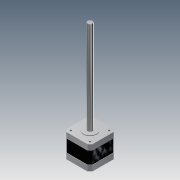
# Autodesk Inventor part: StepperDrive
Saved by Autodesk Inventor 2014 (Build 180170000, 170)
## iProperties
Created: 2014-08-06
Part Number: StepperDrive
Material: Generic
Document SubType Name: Modeling
Designer: Peele
Density: 1 g/cm^3
Appearance: Chrome - Polished
Author: Peele
Autodesk Inventor part; units mm, degrees
ref_plane "YZ Plane" through (0, 0, 0) normal (1, 0, 0) x (0, 1, 0)
ref_plane "XZ Plane" through (0, 0, 0) normal (0, 1, 0) x (-1, 0, 0)
ref_plane "XY Plane" through (0, 0, 0) normal (0, 0, 1) x (1, 0, 0)
sketch "Sketch1" plane through (0, 0, 0) normal (0, 0, 1) x (1, 0, 0)
  line L0 (-21.15, -21.15) -> (21.15, -21.15)
  line L1 (21.15, -21.15) -> (21.15, 21.15)
  line L2 (21.15, 21.15) -> (-21.15, 21.15)
  line L3 (-21.15, 21.15) -> (-21.15, -21.15)
  line L4 (-21.15, -21.15) -> (21.15, 21.15) construction
  line L5 (21.15, -21.15) -> (-21.15, 21.15) construction
  line L6 (-15.5, -15.5) -> (15.5, -15.5) construction
  line L7 (15.5, -15.5) -> (15.5, 15.5) construction
  line L8 (15.5, 15.5) -> (-15.5, 15.5) construction
  line L9 (-15.5, 15.5) -> (-15.5, -15.5) construction
  line L10 (-15.5, -15.5) -> (15.5, 15.5) construction
  line L11 (15.5, -15.5) -> (-15.5, 15.5) construction
  circle A0 centre (-15.5, 15.5) radius 1.5
  circle A1 centre (15.5, 15.5) radius 1.5
  circle A2 centre (15.5, -15.5) radius 1.5
  circle A3 centre (-15.5, -15.5) radius 1.5
  point P0 (0, 0)
  dimension "d0" = 42.3
  dimension "d1" = 31
  dimension "d2" = 3
  constraints: 24 end point, 4 centre point, 4 coincident, 4 midpoint, 4 parallel, 3 equal radius, 3 perpendicular, 2 horizontal, 1 point on line
  measures "d0" distance of L2.end L0.start
  measures "d1" distance of L6.end L7.end
  measures "d2" diameter of A1
extrude "Extrusion1" add sketch "Sketch1" along normal blind 9
chamfer "Chamfer1" distance 4 angle 45 4 edges at (21.15, 21.15, 4.5) (21.15, -21.15, 4.5) (-21.15, 21.15, 4.5) (-21.15, -21.15, 4.5)
sketch "Sketch3" plane through (0, 0, 0) normal (0, 0, -1) x (-1, 0, 0)
  circle A0 centre (15.5, 15.5) radius 1.5 projected
  line L0 (21.15, 17.15) -> (21.15, -17.15) projected
  line L1 (17.15, 21.15) -> (21.15, 17.15) projected
  line L2 (-17.15, 21.15) -> (17.15, 21.15) projected
  line L3 (-21.15, 17.15) -> (-17.15, 21.15) projected
  line L4 (-21.15, -17.15) -> (-21.15, 17.15) projected
  circle A1 centre (15.5, -15.5) radius 1.5 projected
  circle A2 centre (-15.5, -15.5) radius 1.5 projected
  circle A3 centre (-15.5, 15.5) radius 1.5 projected
  circle A4 centre (15.5, 15.5) radius 1.5 projected
  line L5 (21.15, -17.15) -> (17.15, -21.15) projected
  line L6 (21.15, 17.15) -> (21.15, -17.15) projected
  line L7 (17.15, 21.15) -> (21.15, 17.15) projected
  line L8 (-17.15, 21.15) -> (17.15, 21.15) projected
  line L9 (-21.15, 17.15) -> (-17.15, 21.15) projected
  line L10 (-21.15, -17.15) -> (-21.15, 17.15) projected
  line L11 (-17.15, -21.15) -> (-21.15, -17.15) projected
  line L12 (17.15, -21.15) -> (-17.15, -21.15) projected
  line L13 (-20.65, 16.9429) -> (-16.9429, 20.65)
  line L14 (-16.9429, 20.65) -> (16.9429, 20.65)
  line L15 (16.9429, 20.65) -> (20.65, 16.9429)
  line L16 (20.65, 16.9429) -> (20.65, -16.9429)
  line L17 (20.65, -16.9429) -> (16.9429, -20.65)
  line L18 (16.9429, -20.65) -> (-16.9429, -20.65)
  line L19 (-16.9429, -20.65) -> (-20.65, -16.9429)
  line L20 (-20.65, -16.9429) -> (-20.65, 16.9429)
  point P0 (0, 0)
  dimension "d8" = 0.5
  dimension "d10" = 0.5
  dimension "d11" = 0.5
  dimension "d12" = 0.5
  constraints: 16 end point, 4 equal length, 4 parallel, 3 perpendicular, 1 vertical
  measures "d8" distance between parallel lines of L8 L14
  measures "d10" distance between parallel lines of L13 L3
  measures "d11" distance between parallel lines of L4 L20
  measures "d12" distance between parallel lines of L1 L15
extrude "Extrusion2" add sketch "Sketch3" along normal blind 20 contours A0 | A1 | A2 | A3 | L13 L14 L15 L16 L17 L18 L19 L20
sketch "Sketch4" plane through (0, 0, -20) normal (0, 0, -1) x (-1, 0, 0)
  line L0 (-21.15, 17.15) -> (-17.15, 21.15) projected
  line L1 (-17.15, 21.15) -> (17.15, 21.15) projected
  line L2 (17.15, 21.15) -> (21.15, 17.15) projected
  line L3 (21.15, 17.15) -> (21.15, -17.15) projected
  line L4 (21.15, -17.15) -> (17.15, -21.15) projected
  line L5 (17.15, -21.15) -> (-17.15, -21.15) projected
  line L6 (-17.15, -21.15) -> (-21.15, -17.15) projected
  line L7 (-21.15, -17.15) -> (-21.15, 17.15) projected
  point P0 (0, 0)
extrude "Extrusion3" add sketch "Sketch4" along normal blind 9
sketch "Sketch5" plane through (0, 0, 9) normal (0, 0, 1) x (1, 0, 0)
  circle A0 centre (0, 0) radius 11
  dimension "d17" = 22
  constraints: 1 centre point, 1 coincident
  measures "d17" diameter of A0
extrude "Extrusion4" add sketch "Sketch5" along normal blind 1
sketch "Sketch6" plane through (0, 0, 10) normal (0, 0, 1) x (1, 0, 0)
  circle A0 centre (0, 0) radius 11 projected
  circle A1 centre (0, 0) radius 4
  dimension "d20" = 8
  constraints: 1 centre point, 1 coincident
  measures "d20" diameter of A1
extrude "Extrusion5" add sketch "Sketch6" along normal blind 150 contours A1
equation "\"d10\" = d8"
equation "\"d11\" = d8"
equation "\"d12\" = d8"
body "Solid1"
